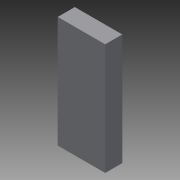
# Autodesk Inventor part: battery pack
Saved by Autodesk Inventor 2015 (Build 190159000, 159)
## iProperties
Created: 2014-09-13
Part Number: battery pack
Material: Generic
Document SubType Name: Modeling
Designer: ericd_000
Density: 1 g/cm^3
Appearance: Default
Author: ericd_000
Autodesk Inventor part; units mm, degrees
ref_plane "YZ Plane" through (0, 0, 0) normal (1, 0, 0) x (0, 1, 0)
ref_plane "XZ Plane" through (0, 0, 0) normal (0, 1, 0) x (-1, 0, 0)
ref_plane "XY Plane" through (0, 0, 0) normal (0, 0, 1) x (1, 0, 0)
sketch "Sketch1" plane through (0, 0, 0) normal (0, 1, 0) x (-1, 0, 0)
  line L0 (51.9761, 72.3524) -> (-6.4439, 72.3524)
  line L1 (-6.4439, 72.3524) -> (-6.4439, -64.8076)
  line L2 (-6.4439, -64.8076) -> (51.9761, -64.8076)
  line L3 (51.9761, -64.8076) -> (51.9761, 72.3524)
  point P0 (0, 0)
  dimension "d0" = 137.16
  dimension "d1" = 58.42
  constraints: 8 end point, 2 parallel, 1 horizontal, 1 perpendicular
  measures "d0" distance of L2.end L0.start
  measures "d1" distance of L0.start L0.end
extrude "Extrusion1" add sketch "Sketch1" along normal blind 21
body "Solid1"
